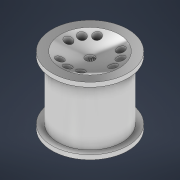
# Autodesk Inventor part: Roda - Estrutura
Saved by Autodesk Inventor 2021 (Build 250183000, 183)
## iProperties
Created: 2021-02-01
Part Number: Roda - Estrutura
Material: Genérico
Document SubType Name: Modeling
Designer: João
Density: 1 g/cm^3
Appearance: Cromado - Polido
Author: João
Autodesk Inventor part; units mm, degrees
sketch "Esboço1" plane through (0, 0, 0) normal (1, 0, 0) x (0, 1, 0)
  line L0 (0, -9) -> (0, -13)
  line L1 (0, -13) -> (1.5, -13)
  line L2 (1.5, -13) -> (1.5, -11)
  line L3 (1.5, -11) -> (21.5, -11)
  line L4 (21.5, -11) -> (21.5, -13)
  line L5 (21.5, -13) -> (23, -13)
  line L6 (23, -13) -> (23, -10)
  line L7 (0, -9) -> (13, -9)
  line L8 (21, -1.5) -> (15.8125, -1.5)
  line L9 (23, 0) -> (0, 0)
  arc A0 (21, -1.5) -> (23, -10) centre (56.4534, 2.3567) ccw
  line L10 (15.9522, -1.5) -> (16.3125, -1.5) construction
  line L11 (13, -3.5) -> (15.5625, -3.5)
  line L12 (13, -3.5) -> (13, -9)
  line L13 (15.5625, -3.5) -> (15.9522, -1.5)
  dimension "d0" = 13
  dimension "d1" = 1.5
  dimension "d2" = 2
  dimension "d3" = 20
  dimension "d4" = 1.5
  dimension "d5" = 13
  constraints: 28 end point, 5 perpendicular, 3 horizontal, 2 point on circle, 2 point on line, 2 vertical, 1 centre point
  measures "d0" distance of L9.end L0.end
  measures "d1" distance of L0.end L1.end
  measures "d2" distance of L1.end L2.end
  measures "d3" distance of L2.end L3.end
  measures "d4" distance of L4.end L5.end
  measures "d5" distance of L0.start L7.end
revolve "Revolução1" add sketch "Esboço1" angle 360 about axis through (0, 23, 0) along (0, -1, 0)
ref_plane "Plano de trabalho1" through (0, 23, 0) normal (0, 1, 0) x (1, 0, 0)
sketch "Esboço3" plane through (0, 23, 0) normal (0, 1, 0) x (1, 0, 0)
  circle A0 centre (0, 0) radius 9 projected
  circle A1 centre (0, 0) radius 9 projected
  circle A2 centre (0, -7.65) radius 1.35
  circle A3 centre (3.5902, -6.7552) radius 1.35
  circle A4 centre (-3.5902, -6.7552) radius 1.35
  circle A5 centre (6.6251, 3.825) radius 1.35
  circle A6 centre (4.0551, 6.4868) radius 1.35
  circle A7 centre (7.6453, 0.2684) radius 1.35
  circle A8 centre (-6.6251, 3.825) radius 1.35
  circle A9 centre (-7.6453, 0.2684) radius 1.35
  circle A10 centre (-4.0551, 6.4868) radius 1.35
  dimension "d34" = 360
  constraints: 9 centre point, 19 other
extrude "Extrusão2" cut sketch "Esboço3" against normal blind 15 contours A5 | A6 | A10 | A8 | A4 | A2 | A3 | A9 | A7
ref_plane "Plano de trabalho2" through (0, 23, -13) normal (0, 0, -1) x (-1, 0, 0)
sketch "Esboço5" plane through (0, 23, -13) normal (0, 0, -1) x (-1, 0, 0)
  line L0 (0, 0) -> (0, -4.5)
  circle A0 centre (0, -4.5) radius 1.5
  point P0 (0, -23)
  dimension "d38" = 4.5
  dimension "d39" = 3
  constraints: 2 end point, 1 centre point, 1 coincident, 1 vertical
  measures "d38" distance of L0.start L0.end
  measures "d39" diameter of A0
extrude "Extrusão3" cut sketch "Esboço5" against normal up to surface
ref_plane "Plano de trabalho3" through (0, 18.5, 0) normal (0, -1, 0) x (1, 0, 0)
sketch "Esboço6" plane through (0, 18.5, 0) normal (0, -1, 0) x (1, 0, 0)
  line L0 (-1.5, -0.25) -> (-1.5, -0.5)
  line L1 (-1.5, -0.25) -> (-1.5, 0)
  circle A0 centre (0, 0) radius 13 projected
  line L2 (0, -0.25) -> (-1.5, -0.25)
  line L3 (-1.5, -10.8972) -> (-1.5, 0) projected
  line L4 (-1.5, -0.25) -> (-2, -0.25)
  line L5 (-2, -0.25) -> (-1.5, -0.5)
  line L6 (-1.5, 0) -> (-2, -0.25)
  line L7 (0, -0.25) -> (0, -0.6278)
  dimension "d45" = 0.25
  dimension "d46" = 0.25
  dimension "d47" = 0.5
  constraints: 14 end point, 2 horizontal, 2 vertical, 1 point on line
  measures "d45" distance of L0.start L0.end
  measures "d46" distance of L0.start L1.end
  measures "d47" distance of L0.start L4.end
coil "Espiral1" sketch "Esboço6" operation cut axis through (0, 18.5, -0.25) along (0, 0, -1) pitch 0.7069 turns 14.5 hand left contours L4 L6 L1 | L0 L5 L4
